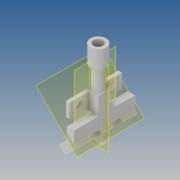
# Autodesk Inventor part: LickSensorMount
Saved by Autodesk Inventor 2020 (Build 240168000, 168)
## iProperties
Created: 2019-07-29
Part Number: LickSensorMount
Material: 일반
Document SubType Name: Modeling
Designer: Jeong Ji Hoon
Density: 1 g/cm^3
Appearance: 기본값
Author: Jeong Ji Hoon
## iProperties of the stored document LickSensorMount_3D 인쇄.ipt
Created: 2019-07-29
Part Number: LickSensorMount_3D 인쇄
Material: 일반
Document SubType Name: Modeling
Designer: Jeong Ji Hoon
Density: 1 g/cm^3
Appearance: 기본값
Author: Jeong Ji Hoon
Autodesk Inventor part; units mm, degrees
ref_plane "YZ Plane" through (0, 0, 0) normal (1, 0, 0) x (0, 1, 0)
ref_plane "XZ Plane" through (0, 0, 0) normal (0, 1, 0) x (-1, 0, 0)
ref_plane "XY Plane" through (0, 0, 0) normal (0, 0, 1) x (1, 0, 0)
sketch "스케치1" plane through (0, 0, 0) normal (0, 1, 0) x (-1, 0, 0)
  line L0 (0, 0) -> (7, 0)
  line L1 (7, 0) -> (7, -7)
  line L2 (7, -7) -> (0, -7)
  line L3 (0, -7) -> (0, 0)
  dimension "d0" = 7
  dimension "d1" = 7
  constraints: 8 end point, 2 parallel, 1 horizontal, 1 perpendicular
  measures "d0" distance of L1.end L2.end
  measures "d1" distance of L0.end L1.end
extrude "돌출1" add sketch "스케치1" along normal blind 10
sketch "스케치2" plane through (0, 10, 0) normal (0, 1, 0) x (1, 0, 0)
  line L0 (-7, 0) -> (0, 0) projected
  line L1 (0, 0) -> (0, 7) projected
  line L2 (0, 7) -> (-7, 7) projected
  line L3 (-7, 7) -> (-7, 0) projected
  circle A0 centre (-3.5, 3.5) radius 3
  line L4 (-7, 3.5) -> (0, 3.5) construction
  line L5 (-3.5, 7) -> (-3.5, 0) construction
  point P0 (-3.5, 3.5)
  dimension "d4" = 6
  constraints: 5 midpoint, 4 end point, 1 centre point, 1 coincident
  measures "d4" diameter of A0
extrude "돌출2" add sketch "스케치2" along normal blind 13 contours A0
sketch "스케치3" plane through (-3.5, 23, -3.5) normal (0, 1, 0) x (1, 0, 0)
  circle A0 centre (0, 0) radius 3 projected
  circle A1 centre (0, 0) radius 4.5
  point P0 (3.5, -3.5)
  dimension "d7" = 9
  constraints: 1 centre point, 1 coincident
  measures "d7" diameter of A1
extrude "돌출3" add sketch "스케치3" along normal blind 10 contours A0 | A1
ref_plane "작업 평면1" through (-3.5, 0, 0) normal (1, 0, 0) x (0, 0, -1)
sketch "스케치4" plane through (-3.5, 0, 0) normal (1, 0, 0) x (0, 0, -1)
  line L0 (8, 33) -> (-1, 33) projected
  line L1 (-1, 23) -> (8, 23) projected
  line L2 (3.5, 33) -> (3.5, 23) construction
  line L3 (3.5, 33) -> (0.75, 33)
  line L4 (0.75, 33) -> (0.75, 28)
  line L5 (0.75, 28) -> (3, 25.5)
  line L6 (3, 25.5) -> (3, 23)
  line L7 (3, 23) -> (3.5, 23)
  line L8 (3.5, 23) -> (3.5, 33)
  point P0 (0, 0)
  dimension "d10" = 2.75
  dimension "d11" = 5
  dimension "d12" = 2.5
  dimension "d13" = 0.5
  constraints: 14 end point, 2 collinear, 2 midpoint, 2 point on line, 1 parallel, 1 vertical
  measures "d10" distance of L2.start L3.end
  measures "d11" distance of L3.end L4.end
  measures "d12" vertical distance of L5.end L4.end
  measures "d13" distance between parallel lines of L6 L2
revolve "회전2" cut sketch "스케치4" angle 360 about axis through (-3.5, 23, -3.5) along (0, 1, 0)
sketch "스케치5" plane through (0, 0, 0) normal (1, 0, 0) x (0, 0, -1)
  line L0 (7, 0) -> (0, 0) projected
  line L1 (-14, -7) -> (21, -7)
  line L2 (21, -7) -> (21, 0)
  line L3 (21, 0) -> (-14, 0)
  line L4 (-14, 0) -> (-14, -7)
  point P0 (3.5, 0)
  dimension "d16" = 35
  dimension "d17" = 7
  constraints: 8 end point, 2 midpoint, 2 parallel, 1 horizontal, 1 perpendicular
  measures "d16" distance of L1.start L1.end
  measures "d17" distance of L3.end L1.start
extrude "돌출4" add sketch "스케치5" against normal blind 4
sketch "스케치6" plane through (0, 0, 0) normal (0, -1, 0) x (1, 0, 0)
  circle A0 centre (-3.5, -3.5) radius 2.5
  circle A1 centre (-3.5, -3.5) radius 4.5 projected
  dimension "d20" = 5
  constraints: 2 coincident, 1 centre point
  measures "d20" diameter of A0
extrude "돌출5" add sketch "스케치6" along normal blind 11 contours A0
ref_plane "작업 평면2" through (0, -7, 0) normal (0.7071068, 0.7071068, 0) x (0, 0, 1)
sketch "스케치7" plane through (0, -7, 0) normal (0.7071068, 0.7071068, 0) x (0, 0, 1)
  line L0 (-7, -4.9497) -> (-7, -12.0208) projected
  line L1 (0, -12.0208) -> (-7, -12.0208) projected
  line L2 (0, -4.9497) -> (0, -12.0208) projected
  line L3 (0, -4.9497) -> (14, -4.9497) projected
  line L4 (14, -4.9497) -> (14, 0) projected
  line L5 (14, 0) -> (-21, 0) projected
  line L6 (-21, 0) -> (-21, -4.9497) projected
  line L7 (-21, -4.9497) -> (-7, -4.9497) projected
  line L8 (-21, 2) -> (14, 2)
  line L9 (14, 2) -> (14, -3)
  line L10 (14, -3) -> (-21, -3)
  line L11 (-21, -3) -> (-21, 2)
  dimension "d23" = 35
  dimension "d24" = 5
  dimension "d25" = 2
  constraints: 8 end point, 2 parallel, 1 collinear, 1 horizontal, 1 perpendicular
  measures "d23" distance of L9.end L10.end
  measures "d24" distance of L8.end L9.end
  measures "d25" distance between parallel lines of L8 L5
extrude "돌출6" add sketch "스케치7" against normal blind 9 contours L6 L5 L4 L10 | L11 L8 L9 L5
sketch "스케치8" plane through (1.4142, -8.4142, 14) normal (0.7071068, -0.7071068, 0) x (-0.7071068, -0.7071068, 0)
  line L0 (0, 35) -> (0, 0) projected
  line L1 (0, 0) -> (9, 0) projected
  line L2 (9, 35) -> (9, 0) projected
  line L3 (0, 35) -> (9, 35) projected
  line L4 (1, 1.5) -> (7, 1.5)
  line L5 (7, 1.5) -> (7, 6.2)
  line L6 (7, 6.2) -> (1, 6.2)
  line L7 (1, 6.2) -> (1, 1.5)
  line L8 (1, 28.8) -> (7, 28.8)
  line L9 (7, 28.8) -> (7, 33.5)
  line L10 (7, 33.5) -> (1, 33.5)
  line L11 (1, 33.5) -> (1, 28.8)
  line L12 (9, 8.2) -> (0, 8.2)
  line L13 (9, 26.8) -> (0, 26.8)
  line L14 (9, 14.7) -> (0, 14.7)
  line L15 (9, 20.3) -> (0, 20.3)
  point P0 (-4.9497, 14)
  dimension "d28" = 6
  dimension "d29" = 4.7
  dimension "d30" = 4.7
  dimension "d31" = 1.5
  dimension "d32" = 2
  dimension "d33" = 1.5
  dimension "d34" = 2
  dimension "d35" = 2
  dimension "d36" = 6.5
  dimension "d37" = 6.5
  constraints: 24 end point, 10 point on line, 5 parallel, 5 perpendicular, 2 horizontal
  measures "d28" distance of L5.end L6.end
  measures "d29" distance of L4.end L5.end
  measures "d30" distance of L8.end L9.end
  measures "d31" distance between parallel lines of L1 L4
  measures "d32" distance between parallel lines of L2 L5
  measures "d33" distance between parallel lines of L3 L10
  measures "d34" distance between parallel lines of L6 L12
  measures "d35" distance between parallel lines of L8 L13
  measures "d36" distance between parallel lines of L12 L14
  measures "d37" distance between parallel lines of L13 L15
extrude "돌출7" cut sketch "스케치8" against normal through all contours L13 L2 L15 L0 | L14 L2 L12 L0 | L7 L6 L5 L4 | L11 L10 L9 L8
sketch "스케치9" plane through (1.4142, -8.4142, -0.7) normal (0.7071068, -0.7071068, 0) x (-0.7071068, -0.7071068, 0)
  line L0 (9, 5.6) -> (9, 0) projected
  line L1 (0, 5.6) -> (0, 0) projected
  line L2 (2, 0.8) -> (7, 0.8)
  line L3 (7, 0.8) -> (7, 4.8)
  line L4 (7, 4.8) -> (2, 4.8)
  line L5 (2, 4.8) -> (2, 0.8)
  line L6 (9, 2.8) -> (0, 2.8) construction
  point P0 (-4.9497, -0.7)
  point P1 (2, 2.8)
  dimension "d40" = 4
  dimension "d41" = 5
  dimension "d42" = 2
  constraints: 10 end point, 3 midpoint, 2 parallel, 1 horizontal, 1 perpendicular, 1 point on line
  measures "d40" distance of L2.end L3.end
  measures "d41" distance of L3.end L4.end
  measures "d42" distance between parallel lines of L3 L0
extrude "돌출8" add sketch "스케치9" along normal blind 2
sketch "스케치10" plane through (2.8284, -9.8284, -0.7) normal (0.7071068, -0.7071068, 0) x (0, 0, -1)
  line L0 (0.8, -2) -> (0.8, -7) projected
  line L1 (0.8, -7) -> (4.8, -7) projected
  line L2 (4.8, -7) -> (4.8, -2) projected
  line L3 (1.05, -4) -> (4.55, -4)
  line L4 (4.55, -4) -> (4.55, -6.5)
  line L5 (4.55, -6.5) -> (1.05, -6.5)
  line L6 (1.05, -6.5) -> (1.05, -4)
  point P0 (-0.7, 4.9497)
  dimension "d45" = 3.5
  dimension "d46" = 2.5
  dimension "d47" = 0.5
  dimension "d48" = 0.25
  dimension "d49" = 0.25
  constraints: 8 end point, 2 parallel, 1 horizontal, 1 perpendicular
  measures "d45" distance of L4.end L5.end
  measures "d46" distance of L3.end L4.end
  measures "d47" distance between parallel lines of L5 L1
  measures "d48" distance between parallel lines of L0 L6
  measures "d49" distance between parallel lines of L2 L4
extrude "돌출9" add sketch "스케치10" along normal blind 2
sketch "스케치11" plane through (4.2426, -11.2426, -0.7) normal (0.7071068, -0.7071068, 0) x (-0.7071068, -0.7071068, 0)
  line L0 (4, 4.55) -> (4, 1.05) projected
  line L1 (4, 1.05) -> (6.5, 1.05) projected
  line L2 (6.5, 1.05) -> (6.5, 4.55) projected
  line L3 (6.5, 4.55) -> (4, 4.55) projected
  line L4 (4.5, 1.55) -> (4.5, 4.05)
  line L5 (4.5, 4.05) -> (6, 4.05)
  line L6 (6, 4.05) -> (6, 1.55)
  line L7 (6, 1.55) -> (4.5, 1.55)
  point P0 (-4.9497, -0.7)
  dimension "d52" = 0.5
  constraints: 8 end point, 3 other
  measures "d52" distance between parallel lines of L0 L4
extrude "돌출10" cut sketch "스케치11" against normal blind 8 contours L4 L5 L6 L7
ref_plane "작업 평면3" through (-7, 10, -3.5) normal (0, 0, 1) x (1, 0, 0)
chamfer "모따기1" distance 1 angle 45 1 edges at (1.4142, -11.2426, -3.5)
sketch "스케치13" plane through (-4, -6.7574, 5.8) normal (0, 0, -1) x (-1, 0, 0)
  line L0 (0, 3.7574) -> (0, 0) projected
  line L1 (0, 0) -> (4.4853, -4.4853) projected
  line L2 (4.4853, -4.4853) -> (0.9497, -8.0208) projected
  line L3 (0.9497, -8.0208) -> (-5.4142, -1.6569) projected
  line L4 (-5.4142, -1.6569) -> (-4, -0.2426) projected
  line L5 (0, 3.7574) -> (-4, -0.2426) projected
  line L6 (0, 6.7574) -> (0, 3.7574) projected
  line L7 (-4, 6.7574) -> (0, 6.7574) projected
  line L8 (-4, -0.2426) -> (-4, 6.7574) projected
  line L9 (0, 0) -> (4.4853, -4.4853) projected
  line L10 (0, 3.7574) -> (0, 0) projected
  line L11 (0, 6.7574) -> (4.4853, -4.4853)
  point P0 (-1.1716, 1.1716)
  point P1 (0, 1.1716)
  constraints: 2 end point
extrude "돌출12" add sketch "스케치13" against normal up to surface (2 mm away) contours L6 L11 L1 L0
sketch "스케치14" plane through (-4, -6.7574, -12.8) normal (0, 0, 1) x (1, 0, 0)
  line L0 (-0.9497, -8.0208) -> (-4.4853, -4.4853) projected
  line L1 (-4.4853, -4.4853) -> (0, 0) projected
  line L2 (0, 0) -> (0, 3.7574) projected
  line L3 (4, -0.2426) -> (0, 3.7574) projected
  line L4 (4, -0.2426) -> (5.4142, -1.6569) projected
  line L5 (5.4142, -1.6569) -> (-0.9497, -8.0208) projected
  line L6 (0, 3.7574) -> (0, 6.7574) projected
  line L7 (0, 6.7574) -> (4, 6.7574) projected
  line L8 (4, 6.7574) -> (4, -0.2426) projected
  line L9 (0, 6.7574) -> (-4.4853, -4.4853)
  constraints: 2 end point
extrude "돌출13" add sketch "스케치14" against normal up to surface (2 mm away) contours L9 L6 L2 L1
sketch "스케치15" plane through (-3.5, 33, -3.5) normal (0, 1, 0) x (1, 0, 0)
  circle A0 centre (0, 0) radius 4.5 projected
  circle A1 centre (0, 0) radius 0.5
  point P0 (3.5, -3.5)
  dimension "d68" = 1
  constraints: 1 centre point, 1 coincident
  measures "d68" diameter of A1
extrude "돌출14" cut sketch "스케치15" against normal up to next contours A1
sketch "스케치16" plane through (-7, 0, 0) normal (-1, 0, 0) x (0, 0, 1)
  line L0 (0, 0) -> (-7, 0) projected
  line L1 (0, 0) -> (0, 10) projected
  line L2 (-7, 10) -> (0, 10) projected
  line L3 (-7, 0) -> (-7, 10) projected
  line L4 (11.5, 10) -> (-18.5, 10)
  line L5 (-18.5, 10) -> (-18.5, 2)
  line L6 (-18.5, 2) -> (11.5, 2)
  line L7 (11.5, 2) -> (11.5, 10)
  point P0 (-3.5, 10)
  dimension "d71" = 30
  dimension "d82" = 8
  constraints: 8 end point, 2 midpoint, 2 parallel, 1 collinear, 1 horizontal, 1 perpendicular
  measures "d71" distance of L5.end L6.end
  measures "d82" distance of L6.end L4.start
extrude "돌출15" add sketch "스케치16" against normal blind 2 contours L1 L4 L7 L6 | L6 L5 L4 L3
sketch "스케치17" plane through (-5, 0, 0) normal (1, 0, 0) x (0, 0, -1)
  line L0 (18.5, 2) -> (18.5, 10) projected
  line L1 (0, 0) -> (7, 0) projected
  line L2 (-11.5, 2) -> (-11.5, 10) projected
  line L3 (-11.5, 10) -> (18.5, 10) projected
  line L4 (18.5, 10) -> (18.5, 2) projected
  circle A0 centre (-5.75, 6) radius 2
  circle A1 centre (12.75, 6) radius 2
  line L5 (0, 0) -> (0, 2) projected
  line L6 (0, 2) -> (-11.5, 2) projected
  line L7 (18.5, 2) -> (7, 2) projected
  line L8 (7, 0) -> (7, 2) projected
  dimension "d74" = 4
  dimension "d75" = 4
  dimension "d76" = 5.75
  dimension "d77" = 5.75
  dimension "d81" = 4
  constraints: 2 centre point, 1 horizontal alignment
  measures "d74" diameter of A0
  measures "d75" diameter of A1
  measures "d76" distance from line of L0 A1.centre
  measures "d77" distance from line of L2 A0.centre
  measures "d81" distance from line of L3 A0.centre
extrude "돌출16" cut sketch "스케치17" against normal through all contours A0 | A1
